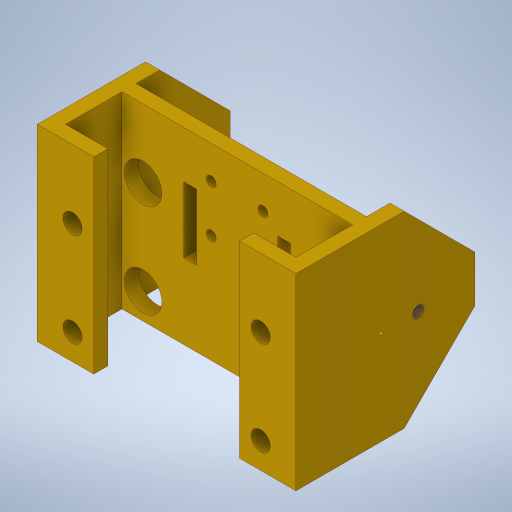
# Autodesk Inventor part: attocube_holder
Saved by Autodesk Inventor 2024 (Build 280153000, 153)
## iProperties
Created: 2021-02-22
Part Number: attocube_holder
Material: Koper
Document SubType Name: Modeling
Designer: rbode
Density: 8.94 g/cm^3
Appearance: Copper - Satin
Author: rbode
Autodesk Inventor part; units mm, degrees
ref_plane "YZ Plane" through (0, 0, 0) normal (1, 0, 0) x (0, 1, 0)
ref_plane "XZ Plane" through (0, 0, 0) normal (0, 1, 0) x (-1, 0, 0)
ref_plane "XY Plane" through (0, 0, 0) normal (0, 0, 1) x (1, 0, 0)
sketch "Sketch1" plane through (0, 0, 0) normal (0, 0, 1) x (1, 0, 0)
  line L0 (27.5, 20) -> (-27.5, 20)
  line L1 (-27.5, 20) -> (-27.5, -20)
  line L2 (-27.5, -20) -> (27.5, -20)
  line L3 (27.5, -20) -> (27.5, 20)
  line L4 (27.5, 20) -> (-27.5, -20) construction
  line L5 (-27.5, 20) -> (27.5, -20) construction
  point P0 (0, 0)
  dimension "d0" = 55
  dimension "d1" = 40
  constraints: 12 end point, 2 midpoint, 2 parallel, 1 horizontal, 1 perpendicular
  measures "d0" distance of L0.start L0.end
  measures "d1" distance of L0.end L1.end
extrude "Extrusion1" add sketch "Sketch1" along normal blind 3
sketch "Sketch2" plane through (0, 0, 3) normal (0, 0, 1) x (1, 0, 0)
  line L0 (27.5, 20) -> (-27.5, 20) projected
  line L1 (-27.5, 20) -> (-27.5, -20) projected
  line L2 (-27.5, -20) -> (27.5, -20) projected
  line L3 (27.5, -20) -> (27.5, 20) projected
  line L4 (-27.5, 20) -> (-24.5, 20)
  line L5 (-24.5, 20) -> (-24.5, -20)
  line L6 (-24.5, -20) -> (-27.5, -20)
  line L7 (-27.5, -20) -> (-27.5, 20)
  line L8 (27.5, 20) -> (24.5, 20)
  line L9 (24.5, 20) -> (24.5, -20)
  line L10 (24.5, -20) -> (27.5, -20)
  line L11 (27.5, -20) -> (27.5, 20)
  point P0 (0, 0)
  dimension "d4" = 3
  dimension "d5" = 3
  constraints: 16 end point, 4 parallel, 2 horizontal, 2 perpendicular, 2 point on line
  measures "d4" distance of L5.end L6.end
  measures "d5" distance of L10.end L9.end
extrude "Extrusion2" add sketch "Sketch2" along normal blind 12 contours L3 L2 L9 L0 | L5 L2 L1 L0
sketch "Sketch3" plane through (0, 0, 15) normal (0, 0, 1) x (1, 0, 0)
  line L0 (-27.5, 20) -> (-27.5, -20) projected
  line L1 (-27.5, -20) -> (-24.5, -20) projected
  line L2 (-24.5, -20) -> (-24.5, 20) projected
  line L3 (-24.5, 20) -> (-27.5, 20) projected
  line L4 (27.5, 20) -> (24.5, 20) projected
  line L5 (24.5, 20) -> (24.5, -20) projected
  line L6 (24.5, -20) -> (27.5, -20) projected
  line L7 (27.5, -20) -> (27.5, 20) projected
  line L8 (-27.5, -20) -> (27.5, -20) projected
  line L9 (-27.5, 20) -> (-15.5, 20)
  line L10 (-15.5, 20) -> (-15.5, -20)
  line L11 (-15.5, -20) -> (-27.5, -20)
  line L12 (-27.5, -20) -> (-27.5, 20)
  line L13 (27.5, 20) -> (15.5, 20)
  line L14 (15.5, 20) -> (15.5, -20)
  line L15 (15.5, -20) -> (27.5, -20)
  line L16 (27.5, -20) -> (27.5, 20)
  point P0 (0, 0)
  dimension "d8" = 12
  dimension "d9" = 12
  constraints: 16 end point, 4 parallel, 2 horizontal, 2 perpendicular, 2 point on line
  measures "d8" distance between parallel lines of L10 L0
  measures "d9" distance between parallel lines of L7 L14
extrude "Extrusion3" add sketch "Sketch3" along normal blind 3
sketch "Sketch4" plane through (0, 0, 18) normal (0, 0, 1) x (1, 0, 0)
  line L0 (-15.5, 20) -> (-27.5, 20) projected
  point P0 (0, 0)
  point P1 (-20, 5.5)
  point P2 (20, 5.5)
  point P3 (20, -14.5)
  point P4 (-20, -14.5)
  dimension "d12" = 40
  dimension "d13" = 20
  dimension "d14" = 14.5
  dimension "d15" = 20
  constraints: 2 horizontal alignment, 2 vertical alignment
  measures "d12" distance of point (20, 5.5) point (-20, 5.5)
  measures "d13" distance of point (-20, -14.5) point (-20, 5.5)
  measures "d14" distance from line of L0 point (-20, 5.5)
  measures "d15" horizontal distance of point (0, 0) point (-20, 5.5)
hole "Hole1" at (-20, 5.5, 18) at (20, 5.5, 18) at (20, -14.5, 18) at (-20, -14.5, 18) direction (0, 0, -1) diameter 4.1 depth 8.8 tip angle 118
sketch "Sketch5" plane through (0, 0, 0) normal (0, 0, -1) x (-1, 0, 0)
  circle A0 centre (20, -14.5) radius 2.05 projected
  circle A1 centre (20, 5.5) radius 2.05 projected
  circle A2 centre (-20, 5.5) radius 2.05 projected
  circle A3 centre (-20, -14.5) radius 2.05 projected
  circle A4 centre (20, -14.5) radius 4
  circle A5 centre (-20, -14.5) radius 2.05 projected
  circle A6 centre (-20, -14.5) radius 4
  circle A7 centre (-20, 5.5) radius 4
  circle A8 centre (20, 5.5) radius 4
  point P0 (0, 0)
  dimension "d23" = 8
  dimension "d24" = 8
  dimension "d25" = 8
  dimension "d26" = 8
  constraints: 4 centre point, 4 coincident
  measures "d23" diameter of A4
  measures "d24" diameter of A6
  measures "d25" diameter of A7
  measures "d26" diameter of A8
extrude "Extrusion4" cut sketch "Sketch5" against normal blind 3 contours A0 | A1 | A2 | A3 | A4 | A6 | A7 | A8
sketch "Sketch6" plane through (0, 0, 0) normal (0, 0, -1) x (-1, 0, 0)
  line L0 (-27.5, 20) -> (27.5, 20) projected
  point P0 (0, 0)
  point P1 (5.5, 3)
  point P2 (-5.5, 3)
  point P3 (-5.5, 13)
  point P4 (5.5, 13)
  dimension "d29" = 5.5
  dimension "d30" = 11
  dimension "d31" = 10
  dimension "d56" = 7
  constraints: 2 horizontal alignment, 2 vertical alignment
  measures "d29" horizontal distance of point (0, 0) point (5.5, 3)
  measures "d30" distance of point (-5.5, 3) point (5.5, 3)
  measures "d31" distance of point (-5.5, 13) point (-5.5, 3)
  measures "d56" distance from line of L0 point (-5.5, 13)
hole "Hole2" at (-5.5, 3, 0) at (5.5, 3, 0) at (5.5, 13, 0) at (-5.5, 13, 0) direction (0, 0, 1) diameter 2.1 depth 8.8 tip angle 118
sketch "Sketch8" plane through (0, 0, 0) normal (0, 0, -1) x (-1, 0, 0)
  line L0 (24.5, 20) -> (24.5, -20) projected
  line L1 (27.5, 20) -> (27.5, -20) projected
  line L2 (-24.5, -20) -> (-24.5, 20) projected
  line L3 (-27.5, -20) -> (-27.5, 20) projected
  line L4 (27.5, -20) -> (24.5, -20)
  line L5 (24.5, -20) -> (24.5, 20)
  line L6 (24.5, 20) -> (27.5, 20)
  line L7 (27.5, 20) -> (27.5, -20)
  line L8 (27.5, -20) -> (-27.5, -20) projected
  line L9 (-27.5, -20) -> (-24.5, -20)
  line L10 (-24.5, -20) -> (-24.5, 20)
  line L11 (-24.5, 20) -> (-27.5, 20)
  line L12 (-27.5, 20) -> (-27.5, -20)
  point P0 (0, 0)
  constraints: 16 end point, 4 parallel, 2 horizontal, 2 perpendicular
extrude "Extrusion5" add sketch "Sketch8" along normal blind 20
sketch "Sketch9" plane through (27.5, -20, 18) normal (1, 0, 0) x (0, 0, -1)
  point P0 (18, 20)
chamfer "Chamfer1" distance 15 angle 45 1 edges at (26, -20, -20)
chamfer "Chamfer2" distance 15 angle 45 3 edges at (26, 20, -20) (-26, -20, -20) (-26, 20, -20)
sketch "Sketch11" plane through (27.5, -20, 18) normal (1, 0, 0) x (0, 0, -1)
  line L0 (38, 25) -> (38, 15) projected
  point P0 (18, 20)
  point P1 (26, 20)
  dimension "d48" = 12
  constraints: 1 horizontal alignment
  measures "d48" distance from line of point (26, 20) L0
hole "Hole3" at (27.5, 0, -8) direction (-1, 0, 0) diameter 2.459 end through all thread size "M3x0.5" class "6H" standard "ANSI Metric M Profile"
sketch "Sketch13" plane through (0, 0, 3) normal (0, 0, 1) x (1, 0, 0)
  line L0 (24.5, 20) -> (-24.5, 20) projected
  point P0 (0, 0)
  point P1 (-10, 1)
  point P2 (10, 1)
  dimension "d57" = 19
  dimension "d58" = 10
  dimension "d59" = 20
  dimension "d60" = 19
  measures "d57" distance from line of L0 point (-10, 1)
  measures "d58" horizontal distance of point (0, 0) point (-10, 1)
  measures "d59" distance of point (-10, 1) point (10, 1)
  measures "d60" distance from line of L0 point (10, 1)
hole "Hole4" at (-10, 1, 3) at (10, 1, 3) direction (0, 0, -1) diameter 2.7 end through all
sketch "Sketch14" plane through (0, 0, 3) normal (0, 0, 1) x (1, 0, 0)
  line L0 (-8.65, -4) -> (-11.35, -4)
  line L1 (-11.35, -4) -> (-11.35, 10)
  line L2 (-11.35, 10) -> (-8.65, 10)
  line L3 (-8.65, 10) -> (-8.65, -4)
  line L4 (-8.65, -4) -> (-11.35, 10) construction
  line L5 (-11.35, -4) -> (-8.65, 10) construction
  line L6 (24.5, 20) -> (-24.5, 20) projected
  line L7 (11.35, 10) -> (8.65, 10)
  line L8 (8.65, 10) -> (8.65, -4)
  line L9 (8.65, -4) -> (11.35, -4)
  line L10 (11.35, -4) -> (11.35, 10)
  point P0 (0, 0)
  point P1 (-10, 3)
  point P2 (-10, 10)
  point P3 (10, 10)
  dimension "d68" = 2.7
  dimension "d69" = 10
  dimension "d70" = 7
  dimension "d71" = 10
  dimension "d72" = 2.7
  dimension "d73" = 10
  dimension "d74" = 14
  dimension "d75" = 10
  constraints: 20 end point, 4 midpoint, 4 parallel, 2 horizontal, 2 perpendicular
  measures "d68" distance of L1.end L2.end
  measures "d69" horizontal distance of point (0, 0) point (-10, 10)
  measures "d70" distance of point (-10, 3) point (-10, 10)
  measures "d71" distance from line of L6 point (-10, 10)
  measures "d72" distance of L9.end L8.end
  measures "d73" distance from line of L6 point (10, 10)
  measures "d74" distance from line of L9 point (10, 10)
  measures "d75" horizontal distance of point (0, 0) point (10, 10)
extrude "Extrusion6" cut sketch "Sketch14" against normal through all
equation "\"d15\" = 0.5 * d12"
equation "\"d29\" = 0.5 * d30"
body "Solid1"
